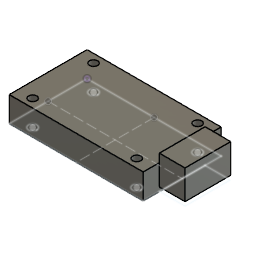
orin_nx_dcdc_v0_1 (Autodesk Fusion 360 design; units mm, degrees)
part number: 2026-05-28-15-44-58-054
Autodesk Fusion 360 part; units mm, degrees
sketch "草图1" plane through (0, 0, 0) normal (0, 1, 0) x (1, 0, 0)
  line L0 (0, 0) -> (60.07, 0)
  line L1 (60.07, 0) -> (60.07, -34.93)
  line L2 (60.07, -34.93) -> (0, -34.93)
  line L3 (0, -34.93) -> (0, 0)
  circle A0 centre (6.72, -3.825) radius 1.84
  circle A1 centre (53.35, -3.825) radius 1.84
  circle A2 centre (53.35, -31.105) radius 1.84
  circle A3 centre (6.72, -31.105) radius 1.84
  line L4 (30.035, 0) -> (30.035, -34.93) construction
  line L5 (0, -17.465) -> (60.07, -17.465) construction
  line L6 (60.07, -7.215) -> (71.57, -7.215)
  line L7 (71.57, -7.215) -> (71.57, -27.715)
  line L8 (71.57, -27.715) -> (60.07, -27.715)
  line L9 (60.07, -27.715) -> (60.07, -7.215)
  point P0 (30.035, 0)
  point P1 (0, -17.465)
  dimension "d1" = 34.93
  dimension "d2" = 60.07
  dimension "d3" = 3.68
  dimension "d4" = 27.28
  dimension "d5" = 46.63
  dimension "d8" = 11.5
  dimension "d9" = 20.5
  constraint horizontal L0
  constraint vertical L1
  constraint horizontal L2
  constraint vertical L3
  constraint coincident L0.start L3.end
  constraint equal A2 A3
  constraint equal A0 A2
  constraint equal A1 A2
  constraint midpoint L0 P0
  constraint midpoint L3 P1
  constraint coincident P0 L4.start
  constraint midpoint L2 L4.end
  constraint coincident P1 L5.start
  constraint midpoint L1 L5.end
  constraint symmetric A2 A3 L4
  constraint symmetric A0 A3 L5
  constraint symmetric A0 A1 L4
  constraint symmetric A1 A2 L5
  constraint horizontal L6
  constraint vertical L7
  constraint horizontal L8
  constraint vertical L9
  constraint coincident L1 L6.start
  constraint symmetric L5 L6.start L8.end
  measures "d1" distance of L0.start L2.end
  measures "d2" distance of L0.start L0.end
  measures "d3" diameter of A2
  measures "d4" distance of A1.centre A2.centre
  measures "d5" distance of A2.centre A3.centre
  measures "d8" distance of L6.start L6.end
  measures "d9" distance of L6.start L8.end
extrude "拉伸1" add sketch "草图1" along normal blind 11.31 contours L0 L1 L2 L3 L9
extrude "拉伸2" add sketch "草图1" along normal blind 15 contours L1 L6 L7 L8 L9
extrude "拉伸3" cut sketch "草图1" along normal blind 1.9 contours L1 L6 L7 L8 L9
